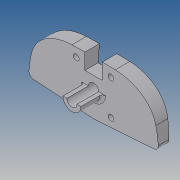
# Autodesk Inventor part: Motormount
Saved by Autodesk Inventor 2019.4 (Build 234330000, 330)
## iProperties
Material: GEDA Stahl
Document SubType Name: Modeling
Designer: Admin
Mass: 172.765 g
Surface Area: 83.2157 cm^2
Volume: 21.9803 cm^3
Density: 7.86 g/cm^3
Appearance: GEDA Stahl A
Gewicht: 0,173 kg
G_L: 0
G_H: 0
G_B: 0
InventorVersion: 2019.4
VAULT_Status: in Bearbeitung
Revision: -
Max. Breite: 0
Max. Höhe: 0
Max. Länge: 0
Max. Abmessungen: 0 x 0 x 0
Author: Admin
Autodesk Inventor part; units mm, degrees
note: some values were not read from the file. Left out: dimensions or parameters whose unit could not be read.
ref_plane "YZ Plane" through (0, 0, 0) normal (1, 0, 0) x (0, 1, 0)
ref_plane "XZ Plane" through (0, 0, 0) normal (0, 1, 0) x (-1, 0, 0)
ref_plane "XY Plane" through (0, 0, 0) normal (0, 0, 1) x (1, 0, 0)
sketch "Skizze1" plane through (0, 0, 0) normal (0, 1, 0) x (-1, 0, 0)
  line L0 (0, -18.5) -> (0, 18.5) construction
  arc A0 (41.721, -15.6557) -> (44.7394, -12.1512) centre (41.5, -12.4133) ccw
  arc A1 (-44.7394, -12.1512) -> (-41.721, -15.6557) centre (-41.5, -12.4133) ccw
  line L1 (0, -18.5) -> (-41.721, -15.6557)
  line L2 (0, -18.5) -> (41.721, -15.6557)
  line L3 (65.5763, 0) -> (-65.5763, 0) projected
  line L4 (-6, 7.5) -> (6, 7.5)
  line L5 (6, 7.5) -> (6, 18.5)
  line L6 (6, 18.5) -> (-6, 18.5) construction
  line L7 (-6, 18.5) -> (-6, 7.5)
  line L8 (-6, 7.5) -> (6, 18.5) construction
  line L9 (6, 7.5) -> (-6, 18.5) construction
  arc A2 (-43.0393, -1) -> (-44.7394, -12.1512) centre (35, -18.603) ccw
  spline S0 degree 3 poles (-43.0393, -1) (-40.2103, 11.542) (-27.2639, 17.9936) (-15, 18.3281) knots 0 0 0 0 1 1 1 1
  arc A3 (44.7394, -12.1512) -> (43.0393, -1) centre (-35, -18.603) ccw
  spline S1 degree 3 poles (15, 18.3281) (27.2639, 17.9936) (40.2103, 11.542) (43.0393, -1) knots 0 0 0 0 1 1 1 1
  arc A4 (15, 18.3281) -> (6, 18.5) centre (0, -531.4673) ccw
  arc A5 (-6, 18.5) -> (-15, 18.3281) centre (0, -531.4673) ccw
  point P0 (0, 0)
  point P1 (0, 0)
  point P2 (0, 13)
  dimension "d3" = 6.5
  dimension "d4" = 3.9
  dimension "d5" = 83
  dimension "d6" = 12
  dimension "d9" = 80
  dimension "d10" = 70
  dimension "d12" = 30
  dimension "d13" = 550
  dimension "d14" = 26
  dimension "d15" = 11
  dimension "d16" = 1
  constraints: 18 end point, 12 point on circle, 6 centre point, 4 midpoint, 4 symmetric about line, 3 tangent, 2 parallel, 1 coincident, 1 equal radius, 1 horizontal, 1 horizontal alignment, 1 perpendicular, 1 point on line, 1 vertical, 10 other
  measures "d3" diameter of A0
  measures "d4" angle of L3 L2
  measures "d5" distance of A0.centre A1.centre
  measures "d6" distance of L6.end L5.end
  measures "d9" radius of A2
  measures "d10" distance of A2.centre A3.centre
  measures "d12" distance of A4.start A5.end
  measures "d13" radius of A5
  measures "d14" distance from line of L0.start L4
  measures "d15" distance of L4.end L5.end
  measures "d16" distance from line of L3 A2.start
extrude "Extrusion1" add sketch "Skizze1" along normal blind 10
sketch "Skizze2" plane through (0, 10, 0) normal (0, 1, 0) x (1, 0, 0)
  circle A0 centre (0, 0.5) radius 3.5
  line L0 (12.0208, 12.5208) -> (-12.0208, 12.5208) construction
  line L1 (-12.0208, 12.5208) -> (-12.0208, -11.5208) construction
  line L2 (-12.0208, -11.5208) -> (12.0208, -11.5208) construction
  line L3 (12.0208, -11.5208) -> (12.0208, 12.5208) construction
  line L4 (12.0208, 12.5208) -> (-12.0208, -11.5208) construction
  line L5 (-12.0208, 12.5208) -> (12.0208, -11.5208) construction
  line L6 (-12.0208, -11.5208) -> (-6.364, -17.1777) construction
  line L7 (12.0208, 12.5208) -> (17.6777, 6.864) construction
  line L8 (12.0208, -11.5208) -> (6.364, -17.1777) construction
  line L9 (-12.0208, 12.5208) -> (-17.6777, 6.864) construction
  circle A1 centre (12.0208, -11.5208) radius 2
  circle A2 centre (-12.0208, -11.5208) radius 2
  circle A3 centre (-12.0208, 12.5208) radius 2
  circle A4 centre (12.0208, 12.5208) radius 2
  point P0 (0, 18.5)
  point P1 (0, 0)
  dimension "d17" = 7
  dimension "d20" = 18
  dimension "d27" = 8
  dimension "d28" = 8
  dimension "d29" = 8
  dimension "d30" = 8
  dimension "d31" = 34
  dimension "d32" = 4
  dimension "d33" = 34
  dimension "d34" = 45
  constraints: 20 end point, 5 centre point, 5 coincident, 3 equal radius, 2 midpoint, 2 parallel, 2 perpendicular, 1 horizontal, 1 vertical alignment
  measures "d17" diameter of A0
  measures "d20" distance of point (0, 18.5) point (0, 0.5)
  measures "d27" distance of L1.end L6.end
  measures "d28" distance of L0.start L7.end
  measures "d29" distance of L2.end L8.end
  measures "d30" distance of L0.end L9.end
  measures "d31" distance between parallel lines of L9 L8
  measures "d32" diameter of A1
  measures "d33" distance between parallel lines of L7 L6
  measures "d34" angle of L4 L2
extrude "Extrusion2" cut sketch "Skizze2" against normal up to next contours A0
sketch "Skizze3" plane through (0, 0, 0) normal (0, -1, 0) x (1, 0, 0)
  circle A0 centre (0, -0.5) radius 3.5 projected
  arc A1 (-6.25, -0.5) -> (6.25, -0.5) centre (0, -0.5) ccw
  line L0 (-6.25, -0.5) -> (-3.5, -0.5)
  circle A2 centre (0, -0.5) radius 3.5 projected
  line L1 (3.5, -0.5) -> (6.25, -0.5)
  point P0 (0, 0)
  dimension "d21" = 12.5
  constraints: 4 end point, 4 point on circle, 3 point on line, 1 centre point, 1 coincident, 1 horizontal
  measures "d21" diameter of A1
extrude "Extrusion3" add sketch "Skizze3" along normal blind 15 contours L1 A1 L0 A0
fillet "Rundung1" radius 2 1 edges at (0, 0, -6.75)
sketch "Skizze5" plane through (0, 0, 0) normal (1, 0, 0) x (0, 1, 0)
  line L0 (10, 18.5) -> (6.7629, -18.5)
  line L1 (6.7629, -18.5) -> (10, -18.5)
  line L2 (10, -18.5) -> (10, 18.5)
  line L3 (10, 3) -> (10, -4) projected
  line L4 (10, -15.6557) -> (10, -18.5) projected
  line L5 (10, -18.5) -> (10, -15.6557) projected
  line L6 (10, -15.6557) -> (10, -12.1512) projected
  line L7 (10, -12.1512) -> (10, -1) projected
  line L8 (10, -1) -> (10, 18.3281) projected
  line L9 (10, 18.3281) -> (10, 18.5) projected
  line L10 (10, 18.5) -> (10, 7.5) projected
  line L11 (10, 7.5) -> (10, 18.5) projected
  line L12 (10, 18.5) -> (10, 18.3281) projected
  line L13 (10, 18.3281) -> (10, -1) projected
  line L14 (10, -1) -> (10, -12.1512) projected
  line L15 (10, -12.1512) -> (10, -15.6557) projected
  point P0 (0, 0)
  dimension "d35" = 5
  constraints: 6 end point, 1 collinear, 1 horizontal, 1 perpendicular
  measures "d35" angle of L2 L0
extrude "Extrusion4" cut sketch "Skizze5" along normal through all both and the other way through all
sketch "Skizze6" plane through (-6, 9.0376, 7.5) normal (0, 0.9962, -0.0872) x (1, 0, 0)
  line L0 (18.0208, 20.0514) -> (-6.0208, 20.0514) construction
  line L1 (-6.0208, 20.0514) -> (-6.0208, -3.9903) construction
  line L2 (-6.0208, -3.9903) -> (18.0208, -3.9903) construction
  line L3 (18.0208, -3.9903) -> (18.0208, 20.0514) construction
  ellipse E0 centre (6, 8.0306) end of major axis (6, 11.5439) minor radius 3.5 projected
  line L4 (18.0208, 20.0514) -> (-6.0208, -3.9903) construction
  line L5 (-6.0208, 20.0514) -> (18.0208, -3.9903) construction
  line L6 (-6.0208, -3.9903) -> (-2.4853, -7.5258) construction
  line L7 (18.0208, 20.0514) -> (21.5563, 16.5158) construction
  circle A0 centre (18.0208, -3.9903) radius 2
  circle A1 centre (-6.0208, -3.9903) radius 2
  circle A2 centre (-6.0208, 20.0514) radius 2
  circle A3 centre (18.0208, 20.0514) radius 2
  point P0 (6, 8.2591)
  dimension "d38" = 45
  dimension "d39" = 5
  dimension "d40" = 5
  dimension "d41" = 34
  dimension "d42" = 4
  constraints: 16 end point, 4 centre point, 4 coincident, 3 equal radius, 2 midpoint, 2 parallel, 2 perpendicular, 1 horizontal, 1 other
  measures "d38" angle of L2 L4
  measures "d39" distance of L1.end L6.end
  measures "d40" distance of L0.start L7.end
  measures "d41" distance between parallel lines of L6 L7
  measures "d42" diameter of A0
extrude "Extrusion5" cut sketch "Skizze6" against normal blind 10 contours A0 | A1 | A2 | A3
equation "\"G_L\" = 0"
equation "\"G_H\" = 0"
equation "\"G_B\" = 0"
